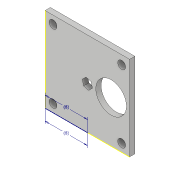
# Autodesk Inventor part: 102
Saved by Autodesk Inventor 2019 (Build 230136000, 136)
## iProperties
Created: 2019-11-17
Part Number: 102
Material: Generic
Document SubType Name: Modeling
Designer: Admin
Density: 1 g/cm^3
Appearance: Default
Author: Admin
Autodesk Inventor part; units mm, degrees
ref_plane "YZ Plane" through (0, 0, 0) normal (1, 0, 0) x (0, 1, 0)
ref_plane "XZ Plane" through (0, 0, 0) normal (0, 1, 0) x (-1, 0, 0)
ref_plane "XY Plane" through (0, 0, 0) normal (0, 0, 1) x (1, 0, 0)
sketch "Sketch1" plane through (0, 0, 0) normal (0, 0, 1) x (1, 0, 0)
  line L0 (0, 0) -> (160, 0)
  line L1 (160, 0) -> (160, 160)
  line L2 (160, 160) -> (0, 160)
  line L3 (0, 160) -> (0, 0)
  dimension "d0" = 160
  dimension "d1" = 160
  constraints: 8 end point, 2 parallel, 1 horizontal, 1 perpendicular
  measures "d0" distance of L2.end L1.end
  measures "d1" distance of L1.end L0.end
extrude "Extrusion1" add sketch "Sketch1" along normal blind 10
sketch "Sketch2" plane through (0, 0, 10) normal (0, 0, 1) x (1, 0, 0)
  line L0 (0, 0) -> (160, 0) projected
  line L1 (0, 0) -> (15, 0)
  line L2 (15, 0) -> (15, 15)
  line L3 (160, 160) -> (0, 160) projected
  line L4 (0, 160) -> (15, 160)
  line L5 (15, 160) -> (15, 145)
  line L6 (160, 0) -> (160, 160) projected
  line L7 (160, 160) -> (145, 160)
  line L8 (145, 160) -> (145, 143.5)
  line L9 (160, 0) -> (160, 15)
  line L10 (160, 15) -> (145, 15)
  circle A0 centre (15, 145) radius 7.5
  circle A1 centre (145, 143.5) radius 7.5
  circle A2 centre (145, 15) radius 7.5
  circle A3 centre (15, 15) radius 7.5
  dimension "d4" = 15
  dimension "d5" = 15
  dimension "d6" = 15
  dimension "d7" = 15
  dimension "d8" = 15
  dimension "d9" = 16.5
  dimension "d10" = 15
  dimension "d11" = 15
  dimension "d12" = 15
  dimension "d13" = 15
  dimension "d14" = 15
  dimension "d15" = 15
  constraints: 16 end point, 4 centre point, 4 coincident, 4 perpendicular, 4 point on line
  measures "d4" distance of L0.start L1.end
  measures "d5" distance of L1.end L2.end
  measures "d6" distance of L3.end L4.end
  measures "d7" distance of L4.end L5.end
  measures "d8" distance of L3.start L7.end
  measures "d9" distance of L7.end L8.end
  measures "d10" distance of L0.end L9.end
  measures "d11" distance of L9.end L10.end
  measures "d12" diameter of A0
  measures "d13" diameter of A1
  measures "d14" diameter of A2
  measures "d15" diameter of A3
extrude "Extrusion2" cut sketch "Sketch2" against normal blind 10
sketch "Sketch3" plane through (0, 0, 10) normal (0, 0, 1) x (1, 0, 0)
  line L0 (0, 160) -> (0, 0) projected
  line L1 (0, 0) -> (80, 0)
  line L2 (0, 0) -> (160, 0) projected
  line L3 (80, 0) -> (0, 0)
  line L4 (0, 0) -> (80, 0)
  dimension "d18" = 80
  dimension "d19" = 80
  dimension "d20" = 80
  constraints: 6 end point, 2 collinear, 1 midpoint
  measures "d18" distance of L0.end L1.end
  measures "d19" distance of L1.end L0.end
  measures "d20" distance of L0.end L1.end
sketch "Sketch4" plane through (0, 0, 10) normal (0, 0, 1) x (1, 0, 0)
  line L0 (0, 0) -> (160, 0) projected
  line L1 (0, 0) -> (0, 80)
  line L2 (0, 160) -> (0, 0) projected
  line L3 (0, 80) -> (80, 80)
  line L4 (87.0711, 87.0711) -> (89.6593, 77.4118)
  line L5 (89.6593, 77.4118) -> (82.5882, 70.3407)
  line L6 (82.5882, 70.3407) -> (72.9289, 72.9289)
  line L7 (72.9289, 72.9289) -> (70.3407, 82.5882)
  line L8 (70.3407, 82.5882) -> (77.4118, 89.6593)
  line L9 (77.4118, 89.6593) -> (87.0711, 87.0711)
  line L10 (160, 0) -> (160, 160) projected
  line L11 (160, 160) -> (160, 80)
  dimension "d21" = 80
  dimension "d22" = 80
  dimension "d23" = 10
  dimension "d24" = 80
  constraints: 18 end point, 2 midpoint, 1 coincident, 1 perpendicular, 13 other
  measures "d21" distance of L0.start L1.end
  measures "d22" distance of L1.end L3.end
  measures "d23" distance of L4.end L5.end
  measures "d24" distance of L10.end L11.end
sketch "Sketch5" plane through (0, 0, 10) normal (0, 0, 1) x (1, 0, 0)
  line L0 (160, 0) -> (160, 160) projected
  line L1 (160, 80) -> (125, 80)
  circle A0 centre (125, 80) radius 29
  point P0 (0, 0)
  dimension "d25" = 35
  dimension "d26" = 58
  constraints: 2 end point, 1 centre point, 1 coincident, 1 horizontal, 1 midpoint
  measures "d25" distance of L1.start L1.end
  measures "d26" diameter of A0
extrude "Extrusion3" cut sketch "Sketch4" against normal blind 10
extrude "Extrusion4" cut sketch "Sketch5" against normal blind 10
body "Solid1"
